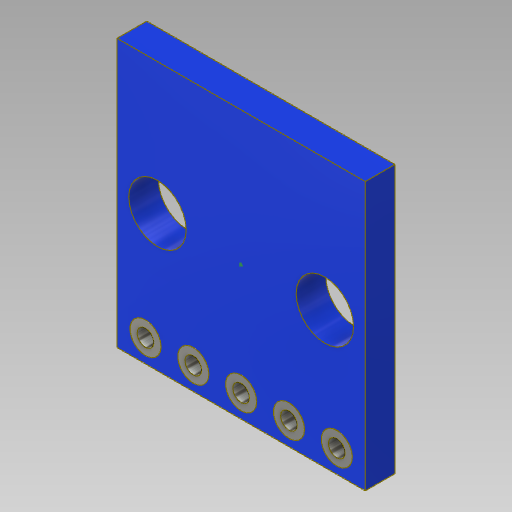
# Autodesk Inventor part: pcb
Saved by Autodesk Inventor 2020 (Build 240168000, 168)
## iProperties
Created: 2018-07-27
Part Number: pcb
Material: Generic
Document SubType Name: Modeling
Designer: amsmi
Density: 1 g/cm^3
Appearance: Default
Author: amsmi
Autodesk Inventor part; units mm, degrees
ref_plane "YZ Plane" through (0, 0, 0) normal (1, 0, 0) x (0, 1, 0)
ref_plane "XZ Plane" through (0, 0, 0) normal (0, 1, 0) x (-1, 0, 0)
ref_plane "XY Plane" through (0, 0, 0) normal (0, 0, 1) x (1, 0, 0)
sketch "Sketch1" plane through (0, 0, 0) normal (0, 0, 1) x (1, 0, 0)
  line L0 (6.5913, -7.112) -> (-6.5913, -7.112)
  line L1 (-6.5913, -7.112) -> (-6.5913, 7.112)
  line L2 (-6.5913, 7.112) -> (6.5913, 7.112)
  line L3 (6.5913, 7.112) -> (6.5913, -7.112)
  line L4 (6.5913, -7.112) -> (-6.5913, 7.112) construction
  line L5 (-6.5913, -7.112) -> (6.5913, 7.112) construction
  point P0 (0, 0)
  dimension "d0" = 13.1826
  dimension "d1" = 14.224
  constraints: 12 end point, 2 midpoint, 2 parallel, 1 horizontal, 1 perpendicular
  measures "d0" distance of L1.end L2.end
  measures "d1" distance of L0.end L1.end
extrude "Extrusion1" add sketch "Sketch1" along normal mid plane 1.5748
sketch "Sketch2" plane through (0, 0, 0.7874) normal (0, 0, 1) x (1, 0, 0)
  circle A0 centre (-4.445, 0.127) radius 1.524
  circle A1 centre (4.445, 0.127) radius 1.524
  line L0 (0, 0) -> (0, 7.112) construction
  line L1 (6.5913, 7.112) -> (-6.5913, 7.112) construction
  dimension "d4" = 3.048
  dimension "d5" = 8.89
  dimension "d6" = 6.985
  constraints: 2 centre point, 2 end point, 1 equal radius, 1 horizontal alignment, 1 midpoint, 1 symmetric about line
  measures "d4" diameter of A0
  measures "d5" distance of A1.centre A0.centre
  measures "d6" distance from line of L1 A0.centre
extrude "Extrusion2" cut sketch "Sketch2" against normal through all
sketch "Sketch3" plane through (0, 0, 0.7874) normal (0, 0, 1) x (1, 0, 0)
  circle A0 centre (0, -5.9055) radius 0.8255 construction
  line L0 (0, -6.731) -> (0, -7.112) construction
  line L1 (6.5913, -7.112) -> (-6.5913, -7.112) construction
  circle A1 centre (-5.08, -5.9055) radius 0.8255
  circle A2 centre (-2.54, -5.9055) radius 0.8255
  circle A3 centre (0, -5.9055) radius 0.8255
  circle A4 centre (2.54, -5.9055) radius 0.8255
  circle A5 centre (5.08, -5.9055) radius 0.8255
  point P0 (0, 0)
  dimension "d9" = 1.651
  dimension "d10" = 0.381
  dimension "d11" = 5.08
  dimension "d14" = 2.54
  constraints: 5 centre point, 2 end point, 2 vertical alignment, 1 horizontal, 1 horizontal alignment, 1 midpoint, 1 vertical, 11 other
  measures "d10" distance of L0.start L0.end
  measures "d11" distance of point (0, -5.906) A1.centre
  measures "d14" distance of A1.centre A2.centre
extrude "Extrusion3" add sketch "Sketch3" along normal blind 0.0025
mirror "Mirror1" about plane through (0, 0, 0) normal (0, 0, 1) of "Extrusion3"
sketch "Sketch4" plane through (-5.08, -5.9055, 0.7899) normal (0, 0, 1) x (1, 0, 0)
  circle A0 centre (0, 0) radius 0.8255 construction
  circle A1 centre (0, 0) radius 0.4445
  circle A2 centre (2.54, 0) radius 0.8255 construction
  line L0 (-1.5113, -1.2065) -> (11.6713, -1.2065) construction
  circle A3 centre (2.54, 0) radius 0.4445
  circle A4 centre (5.08, 0) radius 0.4445
  circle A5 centre (7.62, 0) radius 0.4445
  circle A6 centre (10.16, 0) radius 0.4445
  point P0 (5.08, 5.9055)
  dimension "d21" = 0.889
  dimension "d22" = 2.54
  dimension "d25" = 2.54
  constraints: 5 centre point, 1 coincident, 1 horizontal, 8 other
  measures "d21" diameter of A1
  measures "d22" distance of A2.centre A0.centre
  measures "d25" distance of A1.centre A3.centre
extrude "Extrusion4" cut sketch "Sketch4" against normal through all
sketch "Sketch5" plane through (0, 0, 0.7874) normal (0, 0, 1) x (1, 0, 0)
  point P0 (0, 0)
equation "\"d25\" = d22"
body "Solid1"
